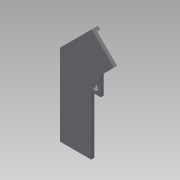
# Autodesk Inventor part: covfronti2c2
Saved by Autodesk Inventor 2015 SP1 (Build 190203100, 203)
## iProperties
Created: 2015-04-15
Part Number: covfronti2c2
Material: Generic
Document SubType Name: Modeling
Designer: Rafi Kurnia Putra
Density: 1 g/cm^3
Appearance: Default
Author: Rafi Kurnia Putra
Autodesk Inventor part; units mm, degrees
ref_plane "YZ Plane" through (0, 0, 0) normal (1, 0, 0) x (0, 1, 0)
ref_plane "XZ Plane" through (0, 0, 0) normal (0, 1, 0) x (-1, 0, 0)
ref_plane "XY Plane" through (0, 0, 0) normal (0, 0, 1) x (1, 0, 0)
sketch "Sketch1" plane through (0, 0, 0) normal (0, 1, 0) x (-1, 0, 0)
  line L0 (25.6659, 82.3437) -> (46.406, 61.6036)
  line L1 (46.406, 61.6036) -> (46.406, 8.9397)
  circle A0 centre (23.593, 50.6893) radius 1.75
  circle A1 centre (23.593, 50.6893) radius 1.75
  line L2 (46.406, 8.9397) -> (26.093, 8.9397)
  line L3 (26.093, 47) -> (19.9037, 47)
  line L4 (19.9037, 47) -> (19.9037, 59.379)
  line L5 (11.3025, 67.9802) -> (19.9037, 59.379)
  line L6 (26.093, 47) -> (26.093, 8.9397)
  line L7 (25.6659, 82.3437) -> (11.3025, 67.9802)
  constraints: 16 end point, 2 centre point
extrude "Extrusion3" add sketch "Sketch1" along normal blind 2
sketch "Sketch3" plane through (0, 2, 0) normal (0, 1, 0) x (1, 0, 0)
  circle A0 centre (-23.593, -50.6893) radius 1.75 projected
  line L0 (-46.406, -8.9397) -> (-46.406, -61.6036) projected
  line L1 (-46.406, -61.6036) -> (-25.6659, -82.3437) projected
  line L2 (-25.6659, -82.3437) -> (-11.3025, -67.9802) projected
  line L3 (-11.3025, -67.9802) -> (-19.9037, -59.379) projected
  line L4 (-19.9037, -59.379) -> (-19.9037, -47) projected
  line L5 (-19.9037, -47) -> (-26.093, -47) projected
  line L6 (-26.093, -47) -> (-26.093, -8.9397) projected
  line L7 (-26.093, -8.9397) -> (-46.406, -8.9397) projected
  line L8 (-46.406, -8.9397) -> (-46.406, -23.9397)
  line L9 (-46.406, -23.9397) -> (-44.406, -23.9397)
  line L10 (-44.406, -23.9397) -> (-44.406, -8.9397)
  line L11 (-44.406, -8.9397) -> (-46.406, -8.9397)
  line L12 (-46.406, -8.9397) -> (-31.406, -8.9397) construction
  line L13 (-46.406, -61.6036) -> (-46.406, -46.6036)
  line L14 (-46.406, -46.6036) -> (-44.406, -46.6036)
  line L15 (-44.406, -46.6036) -> (-44.406, -61.6036)
  line L16 (-44.406, -61.6036) -> (-46.406, -61.6036)
  line L17 (-46.406, -61.6036) -> (-31.406, -61.6036) construction
  line L18 (-46.406, -61.6036) -> (-35.7994, -72.2102)
  line L19 (-35.7994, -72.2102) -> (-34.3852, -70.796)
  line L20 (-34.3852, -70.796) -> (-44.9918, -60.1894)
  line L21 (-44.9918, -60.1894) -> (-46.406, -61.6036)
  line L22 (-46.406, -61.6036) -> (-31.406, -61.6036) construction
  line L23 (-46.406, -61.6036) -> (-25.6659, -82.3437) projected
  line L24 (-25.6659, -82.3437) -> (-30.9692, -77.0404)
  line L25 (-30.9692, -77.0404) -> (-29.555, -75.6262)
  line L26 (-29.555, -75.6262) -> (-24.2517, -80.9295)
  line L27 (-24.2517, -80.9295) -> (-25.6659, -82.3437)
  point P0 (0, 0)
  dimension "d20" = 15
  dimension "d21" = 90
  dimension "d22" = 2
  dimension "d23" = 15
  dimension "d24" = 90
  dimension "d25" = 2
  dimension "d26" = 15
  dimension "d27" = 45
  dimension "d28" = 2
  dimension "d29" = 7.5
  dimension "d30" = 2
  constraints: 38 end point, 8 parallel, 4 perpendicular, 3 collinear, 3 equal length, 3 horizontal, 1 point on line
  measures "d20" distance of L0.start L8.end
  measures "d21" angle of L8 L12
  measures "d22" distance of L9.end L8.end
  measures "d23" distance of L0.end L13.end
  measures "d24" angle of L17 L13
  measures "d25" distance of L13.end L14.end
  measures "d26" distance of L0.end L18.end
  measures "d27" angle of L18 L22
  measures "d28" distance of L19.end L18.end
  measures "d29" distance of L1.end L24.end
  measures "d30" distance of L24.end L25.end
extrude "Extrusion4" add sketch "Sketch3" along normal blind 2 contours L7 L10 L9 L0 | L14 L15 L20 L21 L0 | L16 L15 L20 L19 L1 | L21 L20 L15 L16 | L25 L26 L2 L1
body "Solid2"
